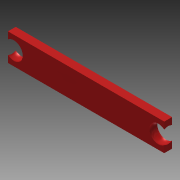
# Autodesk Inventor part: deltabot arm
Saved by Autodesk Inventor 2015 SP2 (Build 190223200, 223)
## iProperties
Created: 2015-05-24
Part Number: deltabot arm
Material: Generic
Document SubType Name: Modeling
Designer: caleb
Density: 1 g/cm^3
Appearance: Light Red
Author: caleb
Autodesk Inventor part; units mm, degrees
ref_plane "YZ Plane" through (0, 0, 0) normal (1, 0, 0) x (0, 1, 0)
ref_plane "XZ Plane" through (0, 0, 0) normal (0, 1, 0) x (-1, 0, 0)
ref_plane "XY Plane" through (0, 0, 0) normal (0, 0, 1) x (1, 0, 0)
sketch "Sketch1" plane through (0, 0, 0) normal (0, 0, 1) x (1, 0, 0)
  line L0 (-50.8, -8.89) -> (50.8, -8.89)
  line L1 (50.8, -8.89) -> (50.8, 8.89)
  line L2 (50.8, 8.89) -> (-50.8, 8.89)
  line L3 (-50.8, 8.89) -> (-50.8, -8.89)
  line L4 (-50.8, -8.89) -> (50.8, 8.89) construction
  line L5 (50.8, -8.89) -> (-50.8, 8.89) construction
  point P0 (0, 0)
  dimension "d18" = 17.78
  dimension "d19" = 101.6
  constraints: 12 end point, 2 midpoint, 2 parallel, 1 horizontal, 1 perpendicular
  measures "d18" distance of L0.end L1.end
  measures "d19" distance of L1.end L2.end
extrude "Extrusion1" add sketch "Sketch1" along normal mid plane 5.08
sketch "Sketch4" plane through (0, 0, 0) normal (0, 0, 1) x (1, 0, 0)
  line L0 (-50.8, -8.89) -> (-50.8, 8.89) construction
  line L1 (-50.8, 8.89) -> (50.8, 8.89) construction
  line L2 (50.8, 8.89) -> (50.8, -8.89) construction
  line L3 (50.8, -8.89) -> (-50.8, -8.89) construction
  arc A0 (46.99, -6.35) -> (46.99, 6.35) centre (46.99, 0) ccw
  line L4 (46.99, 6.35) -> (46.99, -6.35)
  point P0 (0, 0)
  point P1 (50.8, 0)
  dimension "d20" = 6.35
  dimension "d21" = 3.81
  constraints: 2 end point, 2 midpoint, 2 point on circle, 1 centre point, 1 coincident, 1 horizontal alignment, 1 vertical
  measures "d20" radius of A0
  measures "d21" distance between parallel lines of L2 L4
revolve "Revolution2" cut sketch "Sketch4" angle 360 about axis through (46.99, 6.35, 0) along (0, -1, 0)
mirror "Mirror1" about plane through (0, 0, 0) normal (1, 0, 0) of "Revolution2"
body "Solid1"
